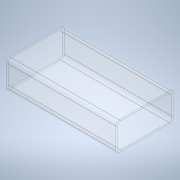
# Autodesk Inventor part: HeatShrink
Saved by Autodesk Inventor 2022 (Build 260153000, 153)
## iProperties
Created: 2022-09-18
Part Number: HeatShrink
Material: Rubber, Silicone
Document SubType Name: Modeling
Designer: Nathan Cai
Density: 1.25 g/cm^3
Appearance: Clear - Light
Author: Nathan Cai
Autodesk Inventor part; units mm, degrees
ref_plane "YZ Plane" through (0, 0, 0) normal (1, 0, 0) x (0, 1, 0)
ref_plane "XZ Plane" through (0, 0, 0) normal (0, 1, 0) x (-1, 0, 0)
ref_plane "XY Plane" through (0, 0, 0) normal (0, 0, 1) x (1, 0, 0)
sketch "Sketch1" plane through (0, 0, 0) normal (1, 0, 0) x (0, 1, 0)
  line L0 (-3.675, 8) -> (3.675, 8)
  line L1 (3.675, 8) -> (3.675, -8)
  line L2 (3.675, -8) -> (-3.675, -8)
  line L3 (-3.675, -8) -> (-3.675, 8)
  line L4 (-3.675, 8) -> (3.675, -8) construction
  line L5 (3.675, 8) -> (-3.675, -8) construction
  line L6 (4.175, -8.5) -> (4.175, 8.5)
  line L7 (4.175, 8.5) -> (-4.175, 8.5)
  line L8 (-4.175, 8.5) -> (-4.175, -8.5)
  line L9 (-4.175, -8.5) -> (4.175, -8.5)
  point P0 (0, 0)
  dimension "d0" = 7.35
  dimension "d1" = 16
  dimension "d2" = 0.5
  constraints: 20 end point, 4 parallel, 2 midpoint, 2 perpendicular, 1 horizontal, 3 other
  measures "d0" distance of L1.end L2.end
  measures "d1" distance of L0.end L1.end
  measures "d2" distance between parallel lines of L1 L6
extrude "Extrusion1" add sketch "Sketch1" along normal blind 28
fillet "Fillet1" radius 1 8 edges at (14, -3.675, -8) (14, 3.675, -8) (14, 4.175, -8.5) (14, 4.175, 8.5) (14, 3.675, 8) (14, -4.175, -8.5) (14, -3.675, 8) (14, -4.175, 8.5)
body "Solid1"
